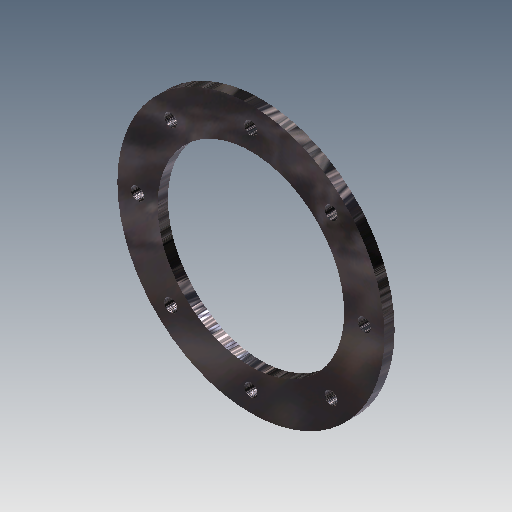
# Autodesk Inventor part: 軸受けワッシャA_ダブルスラスト用(t2_ジュラコン)
Saved by Autodesk Inventor 2019.4 (Build 234330000, 330)
## iProperties
Created: 2018-08-09
Part Number: 軸受けワッシャA_ダブルスラスト用(t2_ジュラコン)
Material: アルミニウム 6061
Document SubType Name: Modeling
Designer: Owner
Density: 2.7 g/cm^3
Appearance: アルミニウム - フラット
Mass: 11.0372 g
Surface Area: 43.3841 cm^2
Volume: 4.08784 cm^3
Author: Owner
Autodesk Inventor part; units mm, degrees
ref_plane "YZ Plane" through (0, 0, 0) normal (1, 0, 0) x (0, 1, 0)
ref_plane "XZ Plane" through (0, 0, 0) normal (0, 1, 0) x (-1, 0, 0)
ref_plane "XY Plane" through (0, 0, 0) normal (0, 0, 1) x (1, 0, 0)
sketch "スケッチ1" plane through (0, 0, 0) normal (0, 0, 1) x (1, 0, 0)
  circle A0 centre (0, 46.1553) radius 11.5 projected
  circle A1 centre (15, 0.6557) radius 1.6 projected
  circle A2 centre (-15, 0.6557) radius 1.6 projected
  circle A3 centre (15, -29.3443) radius 1.6 projected
  circle A4 centre (15, -59.3443) radius 1.6 projected
  circle A5 centre (-15, -29.3443) radius 1.6 projected
  circle A6 centre (-15, -59.3443) radius 1.6 projected
  circle A7 centre (13.5, 17.896) radius 1.1 projected
  circle A8 centre (13.5, 44.896) radius 1.1 projected
  circle A9 centre (-13.5, 17.896) radius 1.1 projected
  circle A10 centre (-13.5, 44.896) radius 1.1 projected
  line L0 (-22.5, 19.3457) -> (-22.5, -66.8443) projected
  line L1 (-22.5, -66.8443) -> (22.5, -66.8443) projected
  line L2 (22.5, -66.8443) -> (22.5, 19.3457) projected
  arc A11 (22.5, 19.3457) -> (-22.5, 19.3457) centre (0, 46.1553) ccw projected
  circle A12 centre (0, 46.1553) radius 5 projected
  circle A13 centre (3.8451, 52.0046) radius 0.8 projected
  circle A14 centre (6.855, 47.5725) radius 0.8 projected
  circle A15 centre (5.8494, 42.3101) radius 0.8 projected
  circle A16 centre (1.4172, 39.3002) radius 0.8 projected
  circle A17 centre (-3.8451, 40.3059) radius 0.8 projected
  circle A18 centre (-6.855, 44.738) radius 0.8 projected
  circle A19 centre (-5.8494, 50.0004) radius 0.8 projected
  circle A20 centre (-1.4172, 53.0103) radius 0.8 projected
  circle A21 centre (0, 46.1553) radius 10 projected
  circle A22 centre (0, 46.1553) radius 32.5
  circle A23 centre (0, 46.1553) radius 22.7
  circle A24 centre (0, 46.1553) radius 22.7 construction
  line L3 (0, 68.8553) -> (0, 78.6553) construction
  circle A25 centre (0, 73.7553) radius 1.6
  circle A26 centre (-19.5161, 65.6714) radius 1.6
  circle A27 centre (-27.6, 46.1553) radius 1.6
  circle A28 centre (-19.5161, 26.6391) radius 1.6
  circle A29 centre (0, 18.5553) radius 1.6
  circle A30 centre (19.5161, 26.6391) radius 1.6
  circle A31 centre (27.6, 46.1553) radius 1.6
  circle A32 centre (19.5161, 65.6714) radius 1.6
  circle A33 centre (0, 46.1553) radius 27.6 construction
  point P0 (0, 0)
  dimension "d0" = 65
  dimension "d1" = 45.4
  dimension "d3" = 3.2
  dimension "d6" = 360
  dimension "d13" = 27.6
  dimension "d14" = 55.2
  constraints: 10 centre point, 2 coincident, 2 end point, 2 vertical alignment, 1 midpoint, 1 vertical, 21 other
  measures "d1" diameter of A23
  measures "d3" diameter of A25
  measures "d13" distance of A0.centre A25.centre
  measures "d14" diameter of A33
extrude "押し出し1" add sketch "スケッチ1" along normal blind 2.5 contours A7 | A9 | A22
